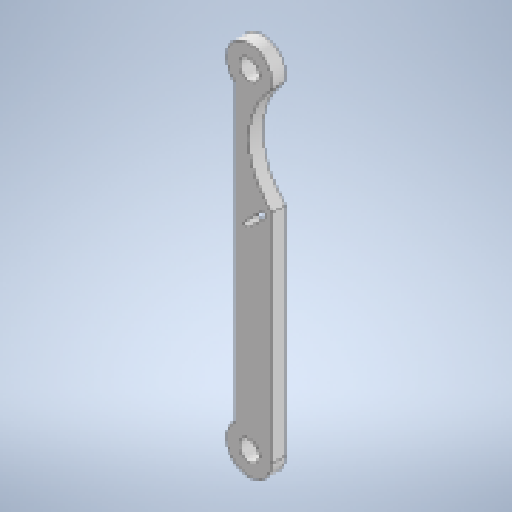
# Autodesk Inventor part: mataroru
Saved by Autodesk Inventor 2024 (Build 280153000, 153)
## iProperties
Created: 2024-06-06
Part Number: mataroru
Material: 一般
Document SubType Name: Modeling
Designer: right
Density: 1 g/cm^3
Appearance: 既定
Author: right
Autodesk Inventor part; units mm, degrees
ref_plane "YZ Plane" through (0, 0, 0) normal (1, 0, 0) x (0, 1, 0)
ref_plane "XZ Plane" through (0, 0, 0) normal (0, 1, 0) x (-1, 0, 0)
ref_plane "XY Plane" through (0, 0, 0) normal (0, 0, 1) x (1, 0, 0)
sketch "スケッチ1" plane through (0, 0, 0) normal (0, 0, 1) x (1, 0, 0)
  line L0 (6.9151, -42.426) -> (18.5151, -42.426) projected
  arc A0 (18.5151, -42.426) -> (22.2151, -40.8167) centre (20.7151, -42.426) ccw projected
  line L1 (22.2151, -40.8167) -> (22.2151, -8.0354) projected
  arc A1 (22.2151, -8.0354) -> (18.9524, -5.1096) centre (20.7151, -6.426) ccw projected
  arc A2 (18.9524, -5.1096) -> (17.3345, -4.0569) centre (12.7151, -12.926) ccw projected
  line L2 (17.3345, -4.0569) -> (8.0957, -4.0569) projected
  arc A3 (8.0957, -4.0569) -> (6.4778, -5.1096) centre (12.7151, -12.926) ccw projected
  arc A4 (6.4778, -5.1096) -> (3.2151, -8.0354) centre (4.7151, -6.426) ccw projected
  line L3 (3.2151, -8.0354) -> (3.2151, -40.8167) projected
  arc A5 (3.2151, -40.8167) -> (6.9151, -42.426) centre (4.7151, -42.426) ccw projected
  circle A6 centre (12.7151, -12.926) radius 6.25 projected
  arc A7 (6.3865, -19.6082) -> (6.0329, -19.2546) centre (6.2097, -19.4314) ccw projected
  line L4 (6.3865, -19.6082) -> (4.6187, -21.3759) projected
  arc A8 (4.2652, -21.0224) -> (4.6187, -21.3759) centre (4.4419, -21.1992) ccw projected
  line L5 (4.2652, -21.0224) -> (6.0329, -19.2546) projected
  arc A9 (9.4254, -21.5214) -> (8.9634, -21.33) centre (9.1944, -21.4257) ccw projected
  line L6 (9.4254, -21.5214) -> (8.4687, -23.8311) projected
  arc A10 (8.0067, -23.6397) -> (8.4687, -23.8311) centre (8.2377, -23.7354) ccw projected
  line L7 (8.0067, -23.6397) -> (8.9634, -21.33) projected
  arc A11 (12.9651, -22.126) -> (12.4651, -22.126) centre (12.7151, -22.126) ccw projected
  line L8 (12.9651, -22.126) -> (12.9651, -24.626) projected
  arc A12 (12.4651, -24.626) -> (12.9651, -24.626) centre (12.7151, -24.626) ccw projected
  line L9 (12.4651, -24.626) -> (12.4651, -22.126) projected
  arc A13 (16.4668, -21.33) -> (16.0048, -21.5214) centre (16.2358, -21.4257) ccw projected
  line L10 (16.4668, -21.33) -> (17.4235, -23.6397) projected
  arc A14 (16.9615, -23.8311) -> (17.4235, -23.6397) centre (17.1925, -23.7354) ccw projected
  line L11 (16.9615, -23.8311) -> (16.0048, -21.5214) projected
  arc A15 (19.3973, -19.2546) -> (19.0437, -19.6082) centre (19.2205, -19.4314) ccw projected
  line L12 (19.3973, -19.2546) -> (21.165, -21.0224) projected
  arc A16 (20.8115, -21.3759) -> (21.165, -21.0224) centre (20.9882, -21.1992) ccw projected
  line L13 (20.8115, -21.3759) -> (19.0437, -19.6082) projected
  circle A17 centre (20.7151, -6.426) radius 0.85 projected
  circle A18 centre (4.7151, -6.426) radius 0.85 projected
  circle A19 centre (4.7151, -42.426) radius 0.85 projected
  circle A20 centre (20.7151, -42.426) radius 0.85 projected
  circle A21 centre (4.7151, -42.426) radius 1.1
  circle A22 centre (4.7151, -6.426) radius 1.1
  circle A23 centre (4.7151, -42.426) radius 2.5
  circle A24 centre (4.7151, -6.426) radius 2.5
  circle A25 centre (12.7151, -12.926) radius 8 projected
  line L14 (7.2151, -42.426) -> (7.2151, -6.426)
  point P0 (0, 0)
  point P1 (3.2151, -40.426)
  point P2 (7.2151, -18.7355)
  point P3 (7.0743, -7.2531)
  point P4 (3.2151, -8.426)
  dimension "d2" = 5
  dimension "d3" = 5
  dimension "d0" = 2.2
  dimension "d1" = 2.2
  constraints: 4 coincident, 2 centre point, 2 end point, 1 point on line, 1 vertical, 6 other
  measures "d0" diameter of A21
  measures "d1" diameter of A22
extrude "押し出し1" add sketch "スケッチ1" along normal blind 1.5 contours A5 L3 A23 L0 | L0 A23 L3 A5 | A23 L3 A24 A25 L14 | A24 A3 A4 L3 | L3 A4 A3 A24 A25 | L4 A8 L5 A7
sketch "スケッチ2" plane through (0, 0, 1.5) normal (0, 0, 1) x (1, 0, 0)
  line L0 (-0.7849, -19.426) -> (2.2151, -19.426)
  line L1 (2.2151, -19.426) -> (2.2151, -29.426)
  line L2 (2.2151, -29.426) -> (-0.7849, -29.426)
  line L3 (-0.7849, -29.426) -> (-0.7849, -19.426)
  line L4 (3.2151, -8.426) -> (3.2151, -40.426) projected
  circle A0 centre (2.2151, -20.526) radius 1.1
  circle A1 centre (-0.7849, -28.326) radius 1.1
  circle A2 centre (2.2151, -28.326) radius 1.1
  circle A3 centre (-0.7849, -20.526) radius 1.1
  line L5 (2.2151, -19.426) -> (3.2151, -19.426)
  line L6 (2.2151, -29.426) -> (3.2151, -29.426)
  line L7 (-1.8849, -20.526) -> (-1.8849, -28.326)
  line L8 (-0.7849, -19.426) -> (-1.8849, -19.426)
  line L9 (-1.8849, -19.426) -> (-1.8849, -20.526)
  line L10 (-0.7849, -29.426) -> (-1.8849, -29.426)
  line L11 (-1.8849, -29.426) -> (-1.8849, -28.326)
  line L12 (-1.8849, -19.426) -> (2.3249, -5.6933)
  arc A4 (7.0743, -7.2531) -> (3.2151, -8.426) centre (4.7151, -6.426) ccw projected
  line L13 (-1.8849, -29.426) -> (2.3249, -43.1587)
  arc A5 (3.2151, -40.426) -> (7.2151, -42.426) centre (4.7151, -42.426) ccw projected
  point P0 (0, 0)
  point P1 (3.2151, -24.426)
  point P2 (2.2151, -24.426)
  point P3 (3.2151, -20.0677)
  point P4 (2.2151, -27.226)
  point P5 (3.2151, -27.8677)
  point P6 (3.2151, -20.9843)
  point P7 (2.2151, -21.626)
  point P8 (3.2151, -28.7843)
  dimension "d8" = 2.2
  dimension "d6" = 3
  dimension "d7" = 10
  dimension "d9" = 1
  constraints: 26 end point, 9 tangent, 7 point on line, 6 point on circle, 3 centre point, 3 perpendicular, 2 horizontal, 2 midpoint, 2 parallel, 1 equal radius, 1 horizontal alignment, 1 vertical, 5 other
  measures "d6" distance of L1.end L2.end
  measures "d7" distance of L0.end L1.end
  measures "d9" distance between parallel lines of L4 L1
extrude "押し出し2" add sketch "スケッチ2" against normal up to surface (1.5 mm away) contours L8 L12 A4 L4 L5 L0 | L5 L4 A0 | A0 L4 A2 L1 | L2 L6 L4 A5 L13 L10 | A2 L4 L6
extrude "押し出し3" cut sketch "スケッチ2" against normal through all contours A0 L4 | A2 L4
